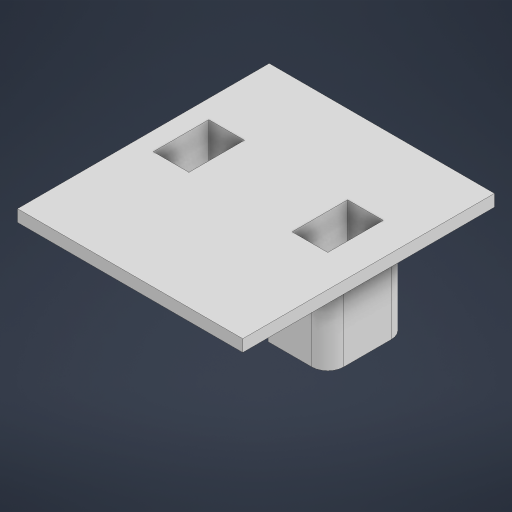
# Autodesk Inventor part: tail_box
Saved by Autodesk Inventor 2024 (Build 280153000, 153)
## iProperties
Created: 2023-05-16
Part Number: tail_box
Material: Типовые
Document SubType Name: Modeling
Designer: user
Density: 1 g/cm^3
Appearance: По умолчанию
Author: user
Autodesk Inventor part; units mm, degrees
ref_plane "YZ Plane" through (0, 0, 0) normal (1, 0, 0) x (0, 1, 0)
ref_plane "XZ Plane" through (0, 0, 0) normal (0, 1, 0) x (-1, 0, 0)
ref_plane "XY Plane" through (0, 0, 0) normal (0, 0, 1) x (1, 0, 0)
sketch "Эскиз1" plane through (0, 0, 0) normal (0, 0, 1) x (1, 0, 0)
  line L0 (0, 0) -> (15, 0)
  line L1 (15, 0) -> (15, 20)
  line L2 (15, 20) -> (0, 20)
  line L3 (0, 20) -> (0, 0)
  line L4 (35, 20) -> (50, 20)
  line L5 (50, 20) -> (50, 0)
  line L6 (50, 0) -> (35, 0)
  line L7 (35, 0) -> (35, 20)
  circle A0 centre (7.5, 10) radius 2
  circle A1 centre (42.5, 10) radius 2
  point P0 (7.5, 20)
  point P1 (15, 10)
  point P2 (35, 10)
  point P3 (42.5, 20)
  dimension "d0" = 4
  dimension "d1" = 15
  dimension "d2" = 20
  dimension "d3" = 20
  constraints: 16 end point, 4 midpoint, 4 parallel, 2 centre point, 2 equal length, 2 horizontal, 2 horizontal alignment, 2 perpendicular, 2 vertical alignment, 1 equal radius, 1 point on line
  measures "d0" diameter of A0
  measures "d1" distance of L1.end L2.end
  measures "d2" distance of L0.end L1.end
  measures "d3" distance of L4.start L1.end
extrude "Выдавливание1" add sketch "Эскиз1" along normal blind 4
sketch "Эскиз2" plane through (0, 0, 4) normal (0, 0, 1) x (1, 0, 0)
  line L0 (15, 0) -> (15, 20) projected
  line L1 (15, 20) -> (0, 20) projected
  line L2 (0, 20) -> (0, 0) projected
  line L3 (0, 0) -> (15, 0) projected
  line L4 (35, 0) -> (50, 0) projected
  line L5 (50, 0) -> (50, 20) projected
  line L6 (50, 20) -> (35, 20) projected
  line L7 (35, 20) -> (35, 0) projected
  line L8 (3, 17) -> (12, 17)
  line L9 (12, 17) -> (12, 3)
  line L10 (12, 3) -> (3, 3)
  line L11 (3, 3) -> (3, 17)
  line L12 (38, 17) -> (47, 17)
  line L13 (47, 17) -> (47, 3)
  line L14 (47, 3) -> (38, 3)
  line L15 (38, 3) -> (38, 17)
  dimension "d6" = 3
  dimension "d7" = 3
  constraints: 16 end point, 6 other
  measures "d6" distance between parallel lines of L1 L8
  measures "d7" distance between parallel lines of L6 L12
extrude "Выдавливание2" add sketch "Эскиз2" along normal blind 17
fillet "Сопряжение1" radius 4 4 edges at (0, 0, 10.5) (50, 0, 10.5) (50, 20, 10.5) (0, 20, 10.5)
sketch "Эскиз3" plane through (0, 0, 21) normal (0, 0, 1) x (1, 0, 0)
  line L0 (-1.6728, 36.9125) -> (55.1159, 36.9125)
  line L1 (55.1159, 36.9125) -> (55.1159, -26.5472)
  line L2 (55.1159, -26.5472) -> (-1.6728, -26.5472)
  line L3 (-1.6728, -26.5472) -> (-1.6728, 36.9125)
  line L4 (3, 17) -> (12, 17) projected
  line L5 (3, 3) -> (3, 17) projected
  line L6 (12, 3) -> (3, 3) projected
  line L7 (12, 17) -> (12, 3) projected
  line L8 (38, 3) -> (38, 17) projected
  line L9 (38, 17) -> (47, 17) projected
  line L10 (47, 17) -> (47, 3) projected
  line L11 (47, 3) -> (38, 3) projected
  point P0 (0, 0)
  constraints: 8 end point, 2 parallel, 1 horizontal, 1 perpendicular
extrude "Выдавливание3" add sketch "Эскиз3" along normal blind 3
